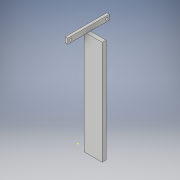
# Autodesk Inventor part: LeftSideTopPlateConnector
Saved by Autodesk Inventor 2017 (Build 210142000, 142)
## iProperties
Created: 2017-12-13
Part Number: LeftSideTopPlateConnector
Material: Generic
Document SubType Name: Modeling
Designer: User
Density: 1 g/cm^3
Appearance: Default
Author: User
Autodesk Inventor part; units mm, degrees
ref_plane "YZ Plane" through (0, 0, 0) normal (1, 0, 0) x (0, 1, 0)
ref_plane "XZ Plane" through (0, 0, 0) normal (0, 1, 0) x (-1, 0, 0)
ref_plane "XY Plane" through (0, 0, 0) normal (0, 0, 1) x (1, 0, 0)
sketch "Sketch1" plane through (0, 0, 0) normal (0, 0, 1) x (1, 0, 0)
  line L0 (0, 0) -> (69.215, 0)
  line L1 (69.215, 0) -> (69.215, -254)
  line L2 (69.215, -254) -> (0, -254)
  line L3 (0, -254) -> (0, 0)
  dimension "d0" = 69.215
  dimension "d1" = 254
  constraints: 8 end point, 2 parallel, 1 horizontal, 1 perpendicular
  measures "d0" distance of L1.end L2.end
  measures "d1" distance of L0.end L1.end
extrude "Extrusion1" add sketch "Sketch1" along normal blind 9.525
sketch "Sketch4" plane through (0, 0, 0) normal (0, 0, -1) x (-1, 0, 0)
  line L0 (-69.215, -254) -> (0, -254) projected
  line L1 (0, 0) -> (-24.765, 0)
  line L2 (-24.765, 0) -> (-24.765, -254)
  line L3 (-24.765, -254) -> (0, -254)
  line L4 (0, -254) -> (0, 0)
  dimension "d11" = 24.765
  constraints: 8 end point, 2 parallel, 1 horizontal, 1 perpendicular, 1 point on line
  measures "d11" distance of L3.end L2.end
extrude "Extrusion4" cut sketch "Sketch4" against normal blind 127
sketch "Sketch5" plane through (69.215, -254, 0) normal (0, -1, 0) x (1, 0, 0)
  point P0 (-69.215, 0)
sketch "Sketch9" plane through (69.215, -254, 0) normal (0, -1, 0) x (1, 0, 0)
  line L0 (-44.45, 9.525) -> (-44.45, 0) projected
  line L1 (0, 0) -> (0, 9.525) projected
  point P0 (-69.215, 0)
  point P1 (-12.7, 4.7625)
  point P2 (-31.75, 4.7625)
hole "Hole2" at (37.465, -254, 4.7625) at (56.515, -254, 4.7625) direction (0, 1, 0) diameter 3.302 depth 7.62 tip angle 118 thread size "8-32 UNC" class "2B" standard "ANSI Unified Screw Threads"
sketch "Sketch11" plane through (69.215, 0, 9.525) normal (0, 1, 0) x (1, 0, 0)
  line L0 (-38.1, -46.0375) -> (-44.45, -46.0375)
  line L1 (-44.45, -46.0375) -> (-44.45, 55.5625)
  line L2 (-44.45, 55.5625) -> (-38.1, 55.5625)
  line L3 (-38.1, 55.5625) -> (-38.1, -46.0375)
  line L4 (-44.45, 9.525) -> (-44.45, 0) projected
  line L5 (0, 0) -> (-44.45, 0) projected
  line L6 (0, 9.525) -> (0, 0) projected
  line L7 (-44.45, 9.525) -> (0, 9.525) projected
  point P0 (-69.215, 9.525)
  dimension "d41" = 6.35
  dimension "d42" = 101.6
  dimension "d44" = 9.525
  dimension "d45" = 46.0375
  dimension "d46" = 0
  constraints: 8 end point, 2 parallel, 1 horizontal, 1 perpendicular
  measures "d41" distance of L1.end L2.end
  measures "d42" distance of L0.end L1.end
  measures "d44" distance of L4.start L4.end
  measures "d45" distance between parallel lines of L7 L2
  measures "d46" distance between parallel lines of L1 L4
extrude "Extrusion7" add sketch "Sketch11" along normal blind 12.7 contours L0 L1 L5 L3 | L5 L1 L7 L3 | L7 L1 L2 L3
sketch "Sketch12" plane through (24.765, -254, 0) normal (-1, 0, 0) x (0, 0, 1)
  line L0 (9.525, 254) -> (9.525, 0) projected
  line L1 (55.5625, 254) -> (9.525, 254) projected
  line L2 (55.5625, 254) -> (55.5625, 266.7) projected
  line L3 (-46.0375, 266.7) -> (55.5625, 266.7) projected
  line L4 (-46.0375, 254) -> (-46.0375, 266.7) projected
  line L5 (0, 254) -> (-46.0375, 254) projected
  line L6 (0, 0) -> (0, 254) projected
  line L7 (9.525, 0) -> (0, 0) projected
  point P0 (-39.6875, 260.35)
  point P1 (49.2125, 260.35)
  dimension "d49" = 12.7
  dimension "d50" = 6.35
  dimension "d51" = 6.35
  dimension "d52" = 6.35
  dimension "d53" = 6.35
  measures "d49" distance of L4.start L3.start
  measures "d50" distance from line of L3 point (-39.687, 260.35)
  measures "d51" distance from line of L4 point (-39.687, 260.35)
  measures "d52" distance from line of L3 point (49.213, 260.35)
  measures "d53" distance from line of L2 point (49.213, 260.35)
hole "Hole3" at (24.765, 6.35, -39.6875) at (24.765, 6.35, 49.2125) direction (1, 0, 0) diameter 6.35 depth 25.4 tip angle 118
equation "\"d45\" = -0.5 * d44 + 0.5 * d42"
equation "\"d50\" = 0.5 * d49"
equation "\"d51\" = d50"
equation "\"d52\" = d50"
equation "\"d53\" = d52"
body "Solid1"
